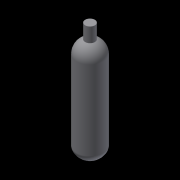
# Autodesk Inventor part: CO2Cartridge16g
Saved by Autodesk Inventor 2020.4 (Build 244396010, 396A)
## iProperties
Created: 2022-09-12
Part Number: CO2Cartridge16g
Material: Generic
Document SubType Name: Modeling
Designer: Val
Density: 1 g/cm^3
Appearance: Default
Author: Val
Autodesk Inventor part; units mm, degrees
ref_plane "YZ Plane" through (0, 0, 0) normal (1, 0, 0) x (0, 1, 0)
ref_plane "XZ Plane" through (0, 0, 0) normal (0, 1, 0) x (-1, 0, 0)
ref_plane "XY Plane" through (0, 0, 0) normal (0, 0, 1) x (1, 0, 0)
sketch "Sketch1" plane through (0, 0, 0) normal (0, 0, 1) x (1, 0, 0)
  line L0 (12.7, 85.09) -> (12.7, 8.89)
  line L1 (12.7, 85.09) -> (0, 85.09)
  line L2 (0, 85.09) -> (0, 8.89)
  line L3 (0, 8.89) -> (12.7, 8.89)
  line L4 (0, 85.09) -> (0, 97.09)
  line L5 (0, 97.09) -> (4.65, 97.09)
  arc A0 (12.7, 85.09) -> (4.65, 97.09) centre (-0.2691, 85.09) ccw
  line L6 (4.65, 97.09) -> (0, 97.09)
  line L7 (0, 97.09) -> (0, 110.806)
  line L8 (0, 110.806) -> (4.65, 110.806)
  line L9 (4.65, 110.806) -> (4.65, 97.09)
  line L10 (0, 8.89) -> (0, 0)
  arc A1 (0, 0) -> (12.7, 8.89) centre (0, 13.5164) ccw
  line L11 (0, 0) -> (12.7, 0)
  line L12 (12.7, 0) -> (12.7, 8.89)
  dimension "d0" = 76.2
  dimension "d1" = 12.7
  dimension "d2" = 12
  dimension "d3" = 4.65
  dimension "d4" = 13.716
  dimension "d5" = 8.89
  constraints: 26 end point, 4 horizontal, 4 point on circle, 4 vertical, 3 perpendicular, 2 centre point, 2 parallel, 2 tangent, 1 coincident, 1 collinear
  measures "d0" distance of L0.start L0.end
  measures "d1" distance of L0.start L1.end
  measures "d2" distance of L1.end L4.end
  measures "d3" distance of L4.end L5.end
  measures "d4" distance of L8.end L5.end
  measures "d5" distance of L2.end L10.end
revolve "Revolution1" add sketch "Sketch1" angle 360 about axis through (0, 85.09, 0) along (0, -1, 0) contours L0 L3 L2 L1 | L1 L4 L5 A0 | A1 L10 L3 | L5 L7 L8 L9
fillet "Fillet1" radius 6 1 edges at (-12.7, 8.89, 0)
body "Solid1"
